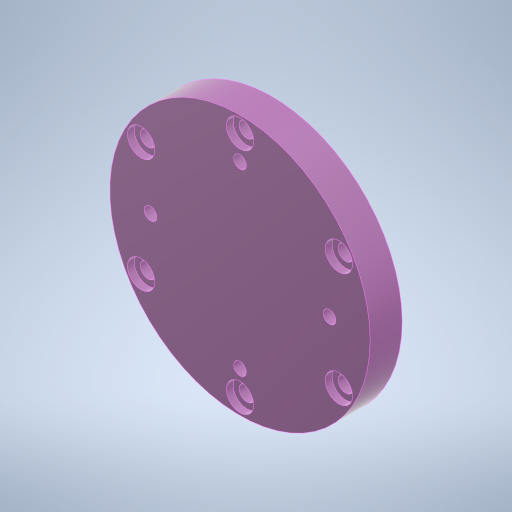
# Autodesk Inventor part: piper-GIM3505-8
Saved by Autodesk Inventor 2024 (Build 280153000, 153)
## iProperties
Created: 2025-04-03
Part Number: piper-GIM3505-8
Material: ABS プラスチック
Document SubType Name: Modeling
Designer: 1412z
Density: 1.06 g/cm^3
Appearance: 滑らか - 紫
Author: 1412z
Autodesk Inventor part; units mm, degrees
ref_plane "YZ Plane" through (0, 0, 0) normal (1, 0, 0) x (0, 1, 0)
ref_plane "XZ Plane" through (0, 0, 0) normal (0, 1, 0) x (-1, 0, 0)
ref_plane "XY Plane" through (0, 0, 0) normal (0, 0, 1) x (1, 0, 0)
sketch "スケッチ1" plane through (0, 0, 0) normal (0, 0, 1) x (1, 0, 0)
  circle A0 centre (0, 0) radius 28.5
  circle A1 centre (0, 0) radius 20
  dimension "d0" = 57
  dimension "d1" = 40
  constraints: 2 centre point, 2 coincident
  measures "d0" diameter of A0
  measures "d1" diameter of A1
extrude "押し出し1" add sketch "スケッチ1" along normal blind 10 contours A0 | A1
sketch "スケッチ2" plane through (0, 0, 0) normal (0, 0, -1) x (-1, 0, 0)
  circle A0 centre (0, 0) radius 22.5
  dimension "d4" = 45
  constraints: 1 centre point, 1 coincident
  measures "d4" diameter of A0
extrude "押し出し2" cut sketch "スケッチ2" against normal blind 5
sketch "スケッチ3" plane through (0, 0, 5) normal (0, 0, -1) x (-1, 0, 0)
  circle A0 centre (0, 0) radius 19.6
  circle A1 centre (19.6, 0) radius 1.4
  circle A2 centre (0, 19.6) radius 1.4
  circle A3 centre (-19.6, 0) radius 1.4
  circle A4 centre (0, -19.6) radius 1.4
  dimension "d7" = 39.2
  dimension "d8" = 2.8
  dimension "d11" = 360
  constraints: 4 centre point, 1 coincident, 1 horizontal alignment, 11 other
  measures "d8" diameter of A1
extrude "押し出し3" cut sketch "スケッチ3" against normal blind 5 contours A0 A1 | A0 A1 | A2 A0 | A0 A2 | A4 A0 | A0 A4 | A3 A0 | A0 A3
sketch "スケッチ4" plane through (0, 0, 10) normal (0, 0, 1) x (1, 0, 0)
  circle A0 centre (0, 0) radius 25
  circle A1 centre (0, -25) radius 1.7
  circle A2 centre (21.6506, -12.5) radius 1.7
  circle A3 centre (21.6506, 12.5) radius 1.7
  circle A4 centre (0, 25) radius 1.7
  circle A5 centre (-21.6506, 12.5) radius 1.7
  circle A6 centre (-21.6506, -12.5) radius 1.7
  dimension "d15" = 50
  dimension "d16" = 3.4
  dimension "d19" = 360
  constraints: 6 centre point, 1 coincident, 1 vertical alignment, 15 other
  measures "d16" diameter of A1
extrude "押し出し4" cut sketch "スケッチ4" against normal blind 10 contours A3 A0 | A0 A3 | A2 A0 | A0 A2 | A4 A0 | A0 A4 | A1 A0 | A0 A1 | A5 A0 | A0 A5 | A6 A0 | A0 A6
sketch "スケッチ5" plane through (0, 0, 10) normal (0, 0, 1) x (1, 0, 0)
  circle A0 centre (0, 0) radius 28.5
  constraints: 1 centre point, 1 coincident
extrude "押し出し5" cut sketch "スケッチ5" against normal blind 3
sketch "スケッチ6" plane through (0, 0, 7) normal (0, 0, 1) x (1, 0, 0)
  circle A0 centre (0, 0) radius 21.5
  circle A1 centre (0, 25) radius 1.7 projected
  circle A2 centre (0, 25) radius 3
  circle A3 centre (-21.6506, 12.5) radius 3
  circle A4 centre (-21.6506, -12.5) radius 3
  circle A5 centre (0, -25) radius 3
  circle A6 centre (21.6506, -12.5) radius 3
  circle A7 centre (21.6506, 12.5) radius 3
  dimension "d25" = 43
  dimension "d26" = 6
  dimension "d29" = 360
  constraints: 7 centre point, 2 coincident, 13 other
  measures "d25" diameter of A0
  measures "d26" diameter of A2
extrude "押し出し6" cut sketch "スケッチ6" against normal blind 1.5 contours A1 | A2 | A3 | A4 | A5 | A6 | A7
